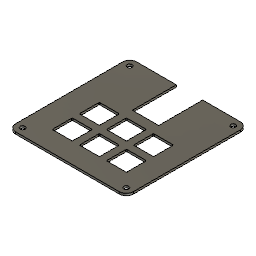
Abhay+Macroboard+Top (Autodesk Fusion 360 design; units mm, degrees)
part number: 2026-01-28-17-49-16-495
Autodesk Fusion 360 part; units mm, degrees
sketch "plate-2026-01-28T23_59_03.859Z" plane through (0, 0, 0) normal (0, 0, 1) x (1, 0, 0)
  line L0 (3.025, -2.525) -> (16.025, -2.525)
  line L1 (3.025, -16.525) -> (16.025, -16.525)
  line L2 (2.525, -3.025) -> (2.525, -16.025)
  line L3 (16.525, -3.025) -> (16.525, -16.025)
  arc A0 (3.025, -2.525) -> (2.525, -3.025) centre (3.025, -3.025) ccw
  arc A1 (16.525, -3.025) -> (16.025, -2.525) centre (16.025, -3.025) ccw
  arc A2 (2.525, -16.025) -> (3.025, -16.525) centre (3.025, -16.025) ccw
  arc A3 (16.025, -16.525) -> (16.525, -16.025) centre (16.025, -16.025) ccw
  line L4 (22.075, -2.525) -> (35.075, -2.525)
  line L5 (22.075, -16.525) -> (35.075, -16.525)
  line L6 (21.575, -3.025) -> (21.575, -16.025)
  line L7 (35.575, -3.025) -> (35.575, -16.025)
  arc A4 (22.075, -2.525) -> (21.575, -3.025) centre (22.075, -3.025) ccw
  arc A5 (35.575, -3.025) -> (35.075, -2.525) centre (35.075, -3.025) ccw
  arc A6 (21.575, -16.025) -> (22.075, -16.525) centre (22.075, -16.025) ccw
  arc A7 (35.075, -16.525) -> (35.575, -16.025) centre (35.075, -16.025) ccw
  line L8 (41.125, -2.525) -> (54.125, -2.525)
  line L9 (41.125, -16.525) -> (54.125, -16.525)
  line L10 (40.625, -3.025) -> (40.625, -16.025)
  line L11 (54.625, -3.025) -> (54.625, -16.025)
  arc A8 (41.125, -2.525) -> (40.625, -3.025) centre (41.125, -3.025) ccw
  arc A9 (54.625, -3.025) -> (54.125, -2.525) centre (54.125, -3.025) ccw
  arc A10 (40.625, -16.025) -> (41.125, -16.525) centre (41.125, -16.025) ccw
  arc A11 (54.125, -16.525) -> (54.625, -16.025) centre (54.125, -16.025) ccw
  line L12 (3.025, -21.575) -> (16.025, -21.575)
  line L13 (3.025, -35.575) -> (16.025, -35.575)
  line L14 (2.525, -22.075) -> (2.525, -35.075)
  line L15 (16.525, -22.075) -> (16.525, -35.075)
  arc A12 (3.025, -21.575) -> (2.525, -22.075) centre (3.025, -22.075) ccw
  arc A13 (16.525, -22.075) -> (16.025, -21.575) centre (16.025, -22.075) ccw
  arc A14 (2.525, -35.075) -> (3.025, -35.575) centre (3.025, -35.075) ccw
  arc A15 (16.025, -35.575) -> (16.525, -35.075) centre (16.025, -35.075) ccw
  line L16 (22.075, -21.575) -> (35.075, -21.575)
  line L17 (22.075, -35.575) -> (35.075, -35.575)
  line L18 (21.575, -22.075) -> (21.575, -35.075)
  line L19 (35.575, -22.075) -> (35.575, -35.075)
  arc A16 (22.075, -21.575) -> (21.575, -22.075) centre (22.075, -22.075) ccw
  arc A17 (35.575, -22.075) -> (35.075, -21.575) centre (35.075, -22.075) ccw
  arc A18 (21.575, -35.075) -> (22.075, -35.575) centre (22.075, -35.075) ccw
  arc A19 (35.075, -35.575) -> (35.575, -35.075) centre (35.075, -35.075) ccw
  line L20 (41.125, -21.575) -> (54.125, -21.575)
  line L21 (41.125, -35.575) -> (54.125, -35.575)
  line L22 (40.625, -22.075) -> (40.625, -35.075)
  line L23 (54.625, -22.075) -> (54.625, -35.075)
  arc A20 (41.125, -21.575) -> (40.625, -22.075) centre (41.125, -22.075) ccw
  arc A21 (54.625, -22.075) -> (54.125, -21.575) centre (54.125, -22.075) ccw
  arc A22 (40.625, -35.075) -> (41.125, -35.575) centre (41.125, -35.075) ccw
  arc A23 (54.125, -35.575) -> (54.625, -35.075) centre (54.125, -35.075) ccw
sketch "Sketch2" plane through (0, 0, 0) normal (0, 0, 1) x (1, 0, 0)
sketch "Sketch3" plane through (0, 0, 0) normal (0, 0, 1) x (1, 0, 0)
  line L0 (-13.96, 35.298) -> (68.953, 35.298)
  line L1 (68.953, 35.298) -> (68.953, -49.996)
  line L2 (68.953, -49.996) -> (-13.96, -49.996)
  line L3 (-13.96, -49.996) -> (-13.96, 35.298)
  circle A0 centre (-8.96, 30.298) radius 1.7
  circle A1 centre (63.953, 30.298) radius 1.7
  circle A2 centre (-8.96, -44.996) radius 1.7
  circle A3 centre (63.953, -44.996) radius 1.7
  line L4 (18.937, 35.298) -> (37.437, 35.298)
  line L5 (37.437, 35.298) -> (37.437, 4.298)
  line L6 (37.437, 4.298) -> (18.937, 4.298)
  line L7 (18.937, 4.298) -> (18.937, 35.298)
  line L8 (2.525, -22.075) -> (2.525, -35.075)
  line L9 (3.025, -35.575) -> (16.025, -35.575)
  dimension "d1" = 82.913
  dimension "d2" = 85.294
  dimension "d5" = 3.4
  dimension "d6" = 3.4
  dimension "d7" = 3.4
  dimension "d8" = 3.4
  dimension "d9" = 5
  dimension "d10" = 5
  dimension "d11" = 5
  dimension "d12" = 5
  dimension "d13" = 5
  dimension "d14" = 5
  dimension "d15" = 5
  dimension "d16" = 5
  dimension "d17" = 18.5
  dimension "d18" = 31
  dimension "d19" = 32.897
  dimension "d26" = 16.485
  dimension "d27" = 14.421
  constraint horizontal L0
  constraint vertical L1
  constraint horizontal L2
  constraint vertical L3
  constraint horizontal L4
  constraint vertical L5
  constraint horizontal L6
  constraint vertical L7
  constraint coincident L0 L4.start
  measures "d1" distance of L0.start L0.end
  measures "d2" distance of L0.start L2.end
  measures "d5" diameter of A0
  measures "d6" diameter of A1
  measures "d7" diameter of A2
  measures "d8" diameter of A3
  measures "d9" distance of L3 A0.centre
  measures "d10" distance of L0 A0.centre
  measures "d11" distance of L1 A1.centre
  measures "d12" distance of L0 A1.centre
  measures "d13" distance of L1 A3.centre
  measures "d14" distance of L2 A3.centre
  measures "d15" distance of L3 A2.centre
  measures "d16" distance of L2 A2.centre
  measures "d17" distance of L4.start L4.end
  measures "d18" distance of L4.start L6.end
  measures "d19" distance of L3 L7
  measures "d26" distance of L3 L8
  measures "d27" distance of L2 L9
sketch "Sketch4" plane through (0, 0, 0) normal (0, 0, 1) x (1, 0, 0)
sketch "Sketch5" plane through (0, 0, 0) normal (0, 0, 1) x (1, 0, 0)
extrude "Extrude1" add sketch "Sketch3" along normal blind 1.5 contours L0 L1 L2 L3 L5 L6 L7
sketch "Sketch6" plane through (0, 0, 1.5) normal (0, 0, 1) x (-1, 0, 0)
  circle A0 centre (-63.953, -30.298) radius 1.7
  circle A1 centre (8.96, 44.996) radius 1.7
  circle A2 centre (-63.953, 44.996) radius 1.7
  circle A3 centre (8.96, -30.298) radius 1.7
  line L0 (-37.437, -35.298) -> (-37.437, -4.298)
  line L1 (-37.437, -4.298) -> (-18.937, -4.298)
  line L2 (-18.937, -4.298) -> (-18.937, -35.298)
  line L3 (-18.937, -35.298) -> (13.96, -35.298)
  line L4 (13.96, -35.298) -> (13.96, 49.996)
  line L5 (13.96, 49.996) -> (-68.953, 49.996)
  line L6 (-68.953, 49.996) -> (-68.953, -35.298)
  line L7 (-68.953, -35.298) -> (-37.437, -35.298)
extrude "Extrude2" cut sketch "plate-2026-01-28T23_59_03.859Z" along normal blind 1.5
fillet "Fillet1" radius 5 4 edges at (-13.96, -49.996, 0.75) (68.953, -49.996, 0.75) (-13.96, 35.298, 0.75) (68.953, 35.298, 0.75)
sketch "Sketch7" plane through (0, 0, 1.5) normal (0, 0, 1) x (-1, 0, 0)
